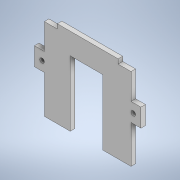
# Autodesk Inventor part: бок
Saved by Autodesk Inventor 2020 (Build 240168000, 168)
## iProperties
Created: 2025-01-18
Part Number: бок
Material: Типовые
Document SubType Name: Modeling
Designer: user
Density: 1 g/cm^3
Appearance: По умолчанию
Author: user
Autodesk Inventor part; units mm, degrees
ref_plane "YZ Plane" through (0, 0, 0) normal (1, 0, 0) x (0, 1, 0)
ref_plane "XZ Plane" through (0, 0, 0) normal (0, 1, 0) x (-1, 0, 0)
ref_plane "XY Plane" through (0, 0, 0) normal (0, 0, 1) x (1, 0, 0)
sketch "Эскиз1" plane through (0, 0, 0) normal (0, 0, 1) x (1, 0, 0)
  line L0 (31.5, -28.5) -> (-31.5, -28.5)
  line L1 (-31.5, -28.5) -> (-31.5, 28.5)
  line L2 (-31.5, 28.5) -> (31.5, 28.5)
  line L3 (31.5, 28.5) -> (31.5, -28.5)
  line L4 (31.5, -28.5) -> (-31.5, 28.5) construction
  line L5 (-31.5, -28.5) -> (31.5, 28.5) construction
  line L6 (-31.5, 28.5) -> (31.5, 28.5)
  line L7 (31.5, 28.5) -> (31.5, 25.5)
  line L8 (31.5, 25.5) -> (-31.5, 25.5)
  line L9 (-31.5, 25.5) -> (-31.5, 28.5)
  line L10 (-31.5, 28.5) -> (-28.5, 28.5)
  line L11 (-28.5, 28.5) -> (-28.5, -28.5)
  line L12 (-28.5, -28.5) -> (-31.5, -28.5)
  line L13 (-31.5, -28.5) -> (-31.5, 28.5)
  line L14 (31.5, 28.5) -> (28.5, 28.5)
  line L15 (28.5, 28.5) -> (28.5, -28.5)
  line L16 (28.5, -28.5) -> (31.5, -28.5)
  line L17 (31.5, -28.5) -> (31.5, 28.5)
  line L18 (11.5, -8.5) -> (-11.5, -8.5)
  line L19 (-11.5, -8.5) -> (-11.5, 14.5)
  line L20 (-11.5, 14.5) -> (11.5, 14.5)
  line L21 (11.5, 14.5) -> (11.5, -8.5)
  line L22 (11.5, -8.5) -> (-11.5, 14.5) construction
  line L23 (-11.5, -8.5) -> (11.5, 14.5) construction
  line L24 (-11.5, 14.5) -> (10, 14.5)
  line L25 (10, 14.5) -> (10, -28.5)
  line L26 (10, -28.5) -> (-11.5, -28.5)
  line L27 (-11.5, -28.5) -> (-11.5, 14.5)
  line L28 (-31.5, 28.5) -> (-28.5, 28.5)
  line L29 (-28.5, 28.5) -> (-28.5, 8.5)
  line L30 (-28.5, 8.5) -> (-31.5, 8.5)
  line L31 (-31.5, 8.5) -> (-31.5, 28.5)
  line L32 (-31.5, 8.5) -> (-28.5, 8.5)
  line L33 (-28.5, 8.5) -> (-28.5, -3.5)
  line L34 (-28.5, -3.5) -> (-31.5, -3.5)
  line L35 (-31.5, -3.5) -> (-31.5, 8.5)
  line L36 (0, 0) -> (0, 3)
  line L37 (28.5, 8.5) -> (31.5, 8.5)
  line L38 (28.5, -3.5) -> (31.5, -3.5)
  line L39 (-20, -22.5) -> (20, -22.5)
  line L40 (20, -22.5) -> (20, 28.5)
  line L41 (20, 28.5) -> (-20, 28.5)
  line L42 (-20, 28.5) -> (-20, -22.5)
  line L43 (-20, -22.5) -> (20, 28.5) construction
  line L44 (20, -22.5) -> (-20, 28.5) construction
  line L45 (-28.5, 2.5) -> (28.5, 2.5)
  line L46 (35, -28.5) -> (-35, -28.5)
  line L47 (-35, -28.5) -> (-35, 28.5)
  line L48 (-35, 28.5) -> (35, 28.5)
  line L49 (35, 28.5) -> (35, -28.5)
  line L50 (35, -28.5) -> (-35, 28.5) construction
  line L51 (-35, -28.5) -> (35, 28.5) construction
  line L52 (-28.5, 2.5) -> (-30, 2.5)
  circle A0 centre (-30, 2.5) radius 1.5
  circle A1 centre (30, 2.5) radius 1.5
  line L53 (-31.5, 8.5) -> (-35, 8.5)
  line L54 (-35, 8.5) -> (-35, -3.5)
  line L55 (-35, -3.5) -> (-31.5, -3.5)
  line L56 (-31.5, -3.5) -> (-31.5, 8.5)
  line L57 (31.5, -3.5) -> (35, -3.5)
  line L58 (35, -3.5) -> (35, 8.5)
  line L59 (35, 8.5) -> (31.5, 8.5)
  line L60 (31.5, 8.5) -> (31.5, -3.5)
  point P0 (-31.5, -3.5)
  point P1 (-11.5, -28.5)
  point P2 (-28.5, 25.5)
  point P3 (-31.5, 8.5)
  point P4 (-20, 25.5)
  point P5 (28.5, -3.5)
  point P6 (31.5, -3.5)
  point P7 (28.5, 8.5)
  point P8 (28.5, 25.5)
  point P9 (20, 25.5)
  point P10 (20, 28.5)
  point P11 (10, -8.5)
  dimension "d0" = 63
  dimension "d1" = 57
  dimension "d2" = 3
  dimension "d3" = 3
  dimension "d4" = 3
  dimension "d5" = 23
  dimension "d6" = 23
  dimension "d7" = 20
  dimension "d8" = 12
  dimension "d12" = 40
  dimension "d13" = 70
  constraints: 122 end point, 24 parallel, 13 horizontal, 13 perpendicular, 10 point on line, 8 midpoint, 6 symmetric about line, 1 centre point, 1 coincident, 1 horizontal alignment, 1 vertical, 3 other
  measures "d0" distance of L1.end L2.end
  measures "d1" distance of L0.end L1.end
  measures "d2" distance of L6.end L7.end
  measures "d3" distance of L11.end L12.end
  measures "d4" distance of L16.end L15.end
  measures "d5" distance of L19.end L20.end
  measures "d6" distance of L18.end L19.end
  measures "d7" distance of L28.end L29.end
  measures "d8" distance of L32.end L33.end
  measures "d12" distance of L41.end L40.end
  measures "d13" distance of L47.end L48.end
extrude "Выдавливание1" add sketch "Эскиз1" along normal blind 3 contours L0 L25 L39 L40 L45 L15 | L38 L15 A1 L3 | L3 L59 L49 L57 | A1 L15 L37 L3 | L0 L11 L45 L42 L39 L27 | L25 L18 L21 L45 L40 L39 | L45 L40 L8 L15 | L39 L42 L45 L19 L27 | L25 L45 L21 L18 | L45 L21 L20 L19 L42 L8 L40 | L34 L1 A0 L11 | L25 L20 L21 L45 | L8 L42 L2 L40 | L55 L47 L53 L1 | A0 L1 L30 L11 | L11 L8 L42 L45
